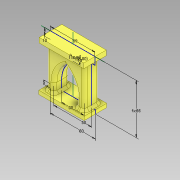
# Autodesk Inventor part: VDPillar_B
Saved by Autodesk Inventor 2021 (Build 250183000, 183)
## iProperties
Created: 2021-03-10
Part Number: VDPillar_B
Material: 一般
Document SubType Name: Modeling
Designer: kumagai
Density: 1 g/cm^3
Appearance: 滑らか - 黄
Author: kumagai
Autodesk Inventor part; units mm, degrees
ref_plane "YZ Plane" through (0, 0, 0) normal (1, 0, 0) x (0, 1, 0)
ref_plane "XZ Plane" through (0, 0, 0) normal (0, 1, 0) x (-1, 0, 0)
ref_plane "XY Plane" through (0, 0, 0) normal (0, 0, 1) x (1, 0, 0)
sketch "スケッチ1" plane through (0, 0, 0) normal (0, 0, 1) x (1, 0, 0)
  line L0 (0, 13.2) -> (0, -79.2)
  line L1 (-42, 0) -> (42, 0)
  line L2 (-30, -66) -> (30, -66)
  line L3 (30, -66) -> (30, -61)
  line L4 (30, -61) -> (-30, -61)
  line L5 (-30, -61) -> (-30, -66)
  line L6 (-10, -61) -> (10, -61)
  line L7 (-29.5, 0) -> (29.5, 0)
  line L8 (29.5, 0) -> (29.5, -10)
  line L9 (29.5, -10) -> (-29.5, -10)
  line L10 (-29.5, -10) -> (-29.5, 0)
  line L11 (-25, -61) -> (-25, -10)
  line L12 (-25, -10) -> (25, -10)
  line L13 (25, -10) -> (25, -61)
  line L14 (-15, -61) -> (-15, -48.814732)
  line L15 (15, -61) -> (15, -48.814732)
  arc A0 (0, -20) -> (-15, -48.814732) centre (20.176292, -48.814732) ccw
  arc A1 (15, -48.814732) -> (0, -20) centre (-20.176292, -48.814732) ccw
  line L16 (7.100794, -15.02797) -> (8.736102, -13.882915)
  line L17 (-5.077891, -16.444422) -> (-6.490474, -15.455321)
  point P0 (0, 0)
  point P1 (30, 0)
  point P2 (25, -10)
  point P3 (-25, -10)
  point P4 (25, -10)
  point P5 (-25, -10)
  dimension "d0" = 60
  dimension "d3" = 5
  dimension "d4" = 10
  dimension "d5" = 59
  dimension "d24" = 66
  dimension "d25" = 50
  dimension "d26" = 30
  dimension "d34" = 10
  dimension "d37" = 110
  dimension "d38" = 35
  constraints: 32 end point, 8 point on line, 4 parallel, 4 perpendicular, 4 point on circle, 4 tangent, 3 horizontal, 3 vertical, 2 centre point, 1 collinear, 1 midpoint, 5 other
  measures "d0" distance between parallel lines of L3 L5
  measures "d3" distance between parallel lines of L2 L4
  measures "d4" distance between parallel lines of L9 L7
  measures "d5" distance between parallel lines of L8 L10
  measures "d24" distance between parallel lines of L2 L7
  measures "d25" distance between parallel lines of L13 L11
  measures "d26" distance between parallel lines of L14 L15
  measures "d34" distance from line of A0.start L12
  measures "d37" angle of L16 L17
  measures "d38" angle of L12 L16
extrude "押し出し1" add sketch "スケッチ1" along normal mid plane 30 contours L4 L3 L2 L0 | L0 L2 L5 L4
extrude "押し出し2" add sketch "スケッチ1" along normal mid plane 20 contours L9 L13 L4 L15 A1 L0 | L0 A0 L14 L4 L11 L9
extrude "押し出し3" add sketch "スケッチ1" along normal mid plane 30 contours L1 L8 L9 L0 | L0 L9 L10 L1
chamfer "面取り7" distance 5 angle 35 4 edges at (29.5, -10, 0) (0, -10, -15) (-29.5, -10, 0) (0, -10, 15)
fillet "フィレット1" radius 4 12 edges at (25, -35.3249, -10) (15, -54.9074, -10) (11.0255, -32.5721, -10) (-15, -54.9074, -10) (-11.0255, -32.5721, -10) (-25, -35.3249, -10) (-25, -35.3249, 10) (-15, -54.9074, 10) (-11.0255, -32.5721, 10) (15, -54.9074, 10) (11.0255, -32.5721, 10) (25, -35.3249, 10)
chamfer "面取り9" distance 3 angle 45 16 edges at (20, -61, -10) (23.8284, -61, -8.8284) (25, -61, 0) (23.8284, -61, 8.8284) (20, -61, 10) (16.1716, -61, 8.8284) (15, -61, 0) (16.1716, -61, -8.8284) (-20, -61, -10) (-16.1716, -61, -8.8284) (-15, -61, 0) (-16.1716, -61, 8.8284) (-20, -61, 10) (-23.8284, -61, 8.8284) (-25, -61, 0) (-23.8284, -61, -8.8284)
equation "\"d24\" = ViaductHeight"
equation "\"ViaductHeight\" = 66"
